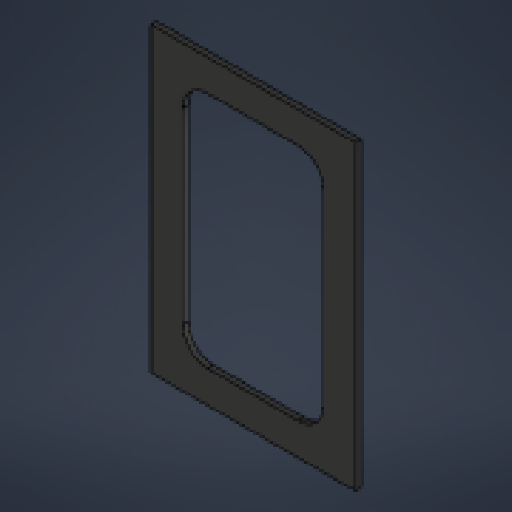
# Autodesk Inventor part: Door Panel Front Foam
Saved by Autodesk Inventor 2026 (Build 300175050, 175E)
## iProperties
Created: 2025-05-22
Part Number: Door Panel Front Foam
Material: Polyurethane Foam
Document SubType Name: Modeling
Designer: Joshua Eah
Density: 0.032 g/cm^3
Appearance: Coarse Textured - Umber
Mass: 7.10468 g
Surface Area: 825.787 cm^2
Volume: 222.021 cm^3
Author: Joshua Eah
Autodesk Inventor part; units mm, degrees
ref_plane "YZ Plane" through (0, 0, 0) normal (1, 0, 0) x (0, 1, 0)
ref_plane "XZ Plane" through (0, 0, 0) normal (0, 1, 0) x (-1, 0, 0)
ref_plane "XY Plane" through (0, 0, 0) normal (0, 0, 1) x (1, 0, 0)
sketch "Sketch1" plane through (0, 0, 0) normal (0, 0, 1) x (1, 0, 0)
  line L0 (0, 0) -> (230, 0)
  line L1 (230, 0) -> (230, 338.262)
  line L2 (230, 338.262) -> (0, 338.262)
  line L3 (0, 338.262) -> (0, 0)
  line L4 (39.012, 39.012) -> (190.988, 39.012)
  line L5 (190.988, 39.012) -> (190.988, 300.162)
  line L6 (190.988, 300.162) -> (39.012, 300.162)
  line L7 (39.012, 300.162) -> (39.012, 39.012)
  dimension "d0" = 230
  dimension "d1" = 338.262
  dimension "d2" = 39.012
  dimension "d3" = 39.012
  dimension "d4" = 39.012
  dimension "d5" = 38.1
  constraints: 16 end point, 4 parallel, 2 horizontal, 2 perpendicular
  measures "d0" distance of L2.end L1.end
  measures "d1" distance of L1.end L0.end
  measures "d2" distance between parallel lines of L0 L4
  measures "d3" distance between parallel lines of L3 L7
  measures "d4" distance between parallel lines of L1 L5
  measures "d5" distance between parallel lines of L2 L6
extrude "Extrusion1" add sketch "Sketch1" along normal blind 6.35
fillet "Fillet2" radius 25.4 4 edges at (190.988, 39.012, 3.175) (39.012, 39.012, 3.175) (39.012, 300.162, 3.175) (190.988, 300.162, 3.175)
thicken "Thicken1" operation add thickness 3 both sides no extend neighbours yes toward (-1, 0, 0) faces at (39.012, 134.5287, 4.2333) (98.1373, 300.162, 2.1167) (190.988, 204.6453, 4.2333) (131.8627, 39.012, 2.1167) (184.2075, 47.1356, 2.1167) (60.6263, 39.2957, 2.1167) (40.7678, 284.0417, 2.1167) (189.2322, 284.0417, 2.1167)
equation "\"d3\" = d2"
equation "\"d4\" = d2"
body "Solid1"
